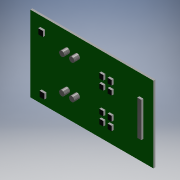
# Autodesk Inventor part: pcb
Saved by Autodesk Inventor 2019.4 (Build 234330000, 330)
## iProperties
Created: 2020-07-10
Part Number: pcb
Material: Generic
Document SubType Name: Modeling
Designer: Jorge
Density: 1 g/cm^3
Appearance: Default
Author: Jorge
Autodesk Inventor part; units mm, degrees
ref_plane "YZ Plane" through (0, 0, 0) normal (1, 0, 0) x (0, 1, 0)
ref_plane "XZ Plane" through (0, 0, 0) normal (0, 1, 0) x (-1, 0, 0)
ref_plane "XY Plane" through (0, 0, 0) normal (0, 0, 1) x (1, 0, 0)
sketch "Sketch1" plane through (0, 0, 0) normal (0, 0, 1) x (1, 0, 0)
  line L0 (151.1214, 28.1918) -> (4.845, 28.1918)
  line L1 (4.845, 28.1918) -> (4.845, -61.9764)
  line L2 (4.845, -61.9764) -> (151.1214, -61.9764)
  line L3 (151.1214, -61.9764) -> (151.1214, 28.1918)
  point P0 (0, 0)
  constraints: 8 end point, 2 parallel, 1 horizontal, 1 perpendicular
extrude "Extrusion1" add sketch "Sketch1" along normal blind 2.5
sketch "Sketch2" plane through (0, 0, 2.5) normal (0, 0, 1) x (1, 0, 0)
  line L0 (16.8135, 16.3028) -> (22.4756, 16.3028)
  line L1 (22.4756, 16.3028) -> (22.4756, 10.0115)
  line L2 (22.4756, 10.0115) -> (16.8135, 10.0115)
  line L3 (16.8135, 10.0115) -> (16.8135, 16.3028)
  line L4 (18.3863, -47.2391) -> (24.0485, -47.2391)
  line L5 (24.0485, -47.2391) -> (24.0485, -53.5303)
  line L6 (24.0485, -53.5303) -> (18.3863, -53.5303)
  line L7 (18.3863, -53.5303) -> (18.3863, -47.2391)
  line L8 (89.3205, 6.7086) -> (94.0389, 6.7086)
  line L9 (94.0389, 6.7086) -> (94.0389, 0.8892)
  line L10 (94.0389, 0.8892) -> (89.3205, 0.8892)
  line L11 (89.3205, 0.8892) -> (89.3205, 6.7086)
  line L12 (99.2282, 6.5498) -> (103.9467, 6.5498)
  line L13 (103.9467, 6.5498) -> (103.9467, 0.7304)
  line L14 (103.9467, 0.7304) -> (99.2282, 0.7304)
  line L15 (99.2282, 0.7304) -> (99.2282, 6.5498)
  line L16 (89.3205, -4.037) -> (94.0389, -4.037)
  line L17 (94.0389, -4.037) -> (94.0389, -9.4978)
  line L18 (94.0389, -9.4978) -> (89.3205, -9.4978)
  line L19 (89.3205, -9.4978) -> (89.3205, -4.037)
  line L20 (99.2282, -4.037) -> (103.9467, -4.037)
  line L21 (103.9467, -4.037) -> (103.9467, -9.5401)
  line L22 (103.9467, -9.5401) -> (99.2282, -9.5401)
  line L23 (99.2282, -9.5401) -> (99.2282, -4.037)
  line L24 (134.3826, 3.7989) -> (139.3028, 3.7989)
  line L25 (139.3028, 3.7989) -> (139.3028, -37.6548)
  line L26 (139.3028, -37.6548) -> (134.3826, -37.6548)
  line L27 (134.3826, -37.6548) -> (134.3826, 3.7989)
  line L28 (89.3205, -30.3157) -> (94.0389, -30.3157)
  line L29 (94.0389, -30.3157) -> (94.0389, -35.7312)
  line L30 (94.0389, -35.7312) -> (89.3205, -35.7312)
  line L31 (89.3205, -35.7312) -> (89.3205, -30.3157)
  line L32 (99.2282, -30.3157) -> (103.9467, -30.3157)
  line L33 (103.9467, -30.3157) -> (103.9467, -36.3609)
  line L34 (103.9467, -36.3609) -> (99.2282, -36.3609)
  line L35 (99.2282, -36.3609) -> (99.2282, -30.3157)
  line L36 (99.2282, -40.517) -> (103.9467, -40.517)
  line L37 (103.9467, -40.517) -> (103.9467, -46.1844)
  line L38 (103.9467, -46.1844) -> (99.2282, -46.1844)
  line L39 (99.2282, -46.1844) -> (99.2282, -40.517)
  line L40 (89.3205, -40.517) -> (94.0614, -40.517)
  line L41 (94.0614, -40.517) -> (94.0614, -46.1844)
  line L42 (94.0614, -46.1844) -> (89.3205, -46.1844)
  line L43 (89.3205, -46.1844) -> (89.3205, -40.517)
  point P0 (0, 0)
  constraints: 88 end point, 22 parallel, 11 horizontal, 11 perpendicular, 7 point on line
extrude "Extrusion2" add sketch "Sketch2" along normal blind 2.5
sketch "Sketch3" plane through (0, 0, 2.5) normal (0, 0, 1) x (1, 0, 0)
  circle A0 centre (48.9712, 8.1491) radius 3.1363
  circle A1 centre (60.8345, 8.1491) radius 3.1363
  circle A2 centre (48.9712, -32.3541) radius 3.1454
  circle A3 centre (60.8345, -32.3541) radius 3.1363
  point P0 (0, 0)
  constraints: 4 centre point
extrude "Extrusion3" add sketch "Sketch3" along normal blind 6.75
body "Solid1"
